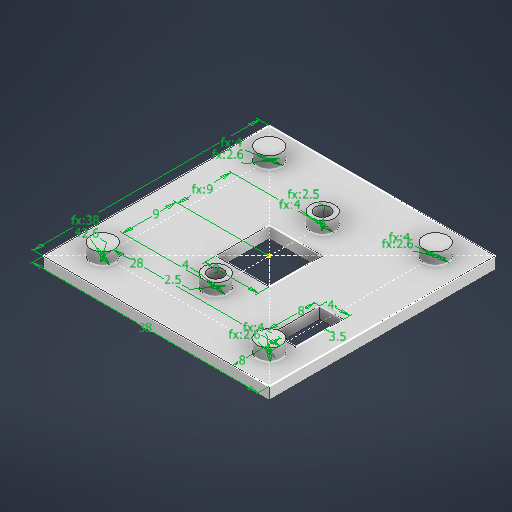
# Autodesk Inventor part: CameraMount
Saved by Autodesk Inventor 2025.1 (Build 291241000, 241)
## iProperties
Created: 2024-11-09
Part Number: CameraMount
Material: Generic
Document SubType Name: Modeling
Designer: jerem
Density: 1 g/cm^3
Appearance: Default
Author: jerem
## iProperties of the stored document CameraMount_3DPrint.ipt
Created: 2024-11-09
Part Number: CameraMount_3DPrint
Material: Generic
Document SubType Name: Modeling
Designer: jerem
Density: 1 g/cm^3
Appearance: Default
Author: jerem
Autodesk Inventor part; units mm, degrees
ref_plane "YZ Plane" through (0, 0, 0) normal (1, 0, 0) x (0, 1, 0)
ref_plane "XZ Plane" through (0, 0, 0) normal (0, 1, 0) x (-1, 0, 0)
ref_plane "XY Plane" through (0, 0, 0) normal (0, 0, 1) x (1, 0, 0)
sketch "Sketch1" plane through (0, 0, 0) normal (0, 1, 0) x (-1, 0, 0)
  line L0 (-19, -19) -> (19, -19)
  line L1 (19, -19) -> (19, 19)
  line L2 (19, 19) -> (-19, 19)
  line L3 (-19, 19) -> (-19, -19)
  line L4 (-19, -19) -> (19, 19) construction
  line L5 (19, -19) -> (-19, 19) construction
  line L6 (4.5, -4.5) -> (-4.5, -4.5)
  line L7 (-4.5, -4.5) -> (-4.5, 4.5)
  line L8 (-4.5, 4.5) -> (4.5, 4.5)
  line L9 (4.5, 4.5) -> (4.5, -4.5)
  line L10 (4.5, -4.5) -> (-4.5, 4.5) construction
  line L11 (-4.5, -4.5) -> (4.5, 4.5) construction
  circle A0 centre (14, 14) radius 1.3
  circle A1 centre (0, 9) radius 1.25
  circle A2 centre (-14, 14) radius 1.3
  circle A3 centre (0, -9) radius 1.25
  line L12 (0, 0) -> (0, 9) construction
  line L13 (0, -9) -> (0, 0) construction
  circle A4 centre (14, -14) radius 1.3
  circle A5 centre (-14, -14) radius 1.3
  line L14 (14, 14) -> (14, -14) construction
  line L15 (14, 14) -> (-14, 14) construction
  line L16 (-14, 14) -> (-14, -14) construction
  circle A6 centre (0, -9) radius 2
  circle A7 centre (0, 9) radius 2
  circle A8 centre (14, 14) radius 2
  circle A9 centre (-14, 14) radius 2
  circle A10 centre (-14, -14) radius 2
  circle A11 centre (14, -14) radius 2
  line L17 (-11.5, 3) -> (-15.5, 3)
  line L18 (-15.5, 3) -> (-15.5, 11)
  line L19 (-15.5, 11) -> (-11.5, 11)
  line L20 (-11.5, 11) -> (-11.5, 3)
  point P0 (0, 0)
  dimension "d0" = 38
  dimension "d1" = 38
  dimension "d2" = 9
  dimension "d3" = 2.5
  dimension "d4" = 2.5
  dimension "d5" = 9
  dimension "d6" = 9
  dimension "d7" = 2.6
  dimension "d8" = 2.6
  dimension "d9" = 2.6
  dimension "d10" = 2.6
  dimension "d11" = 28
  dimension "d14" = 4
  dimension "d15" = 4
  dimension "d16" = 4
  dimension "d17" = 4
  dimension "d18" = 4
  dimension "d19" = 4
  dimension "d20" = 8
  dimension "d21" = 4
  dimension "d22" = 8
  dimension "d23" = 3.5
  constraints: 43 end point, 12 centre point, 7 coincident, 6 parallel, 5 point on line, 4 horizontal, 4 midpoint, 4 vertical, 3 perpendicular
  measures "d0" distance of L3.start L4.end
  measures "d1" distance of L0.end L4.end
  measures "d2" distance of L7.end L8.end
  measures "d3" diameter of A1
  measures "d4" diameter of A3
  measures "d5" distance of L13.end L13.start
  measures "d6" distance of L13.end L12.end
  measures "d7" diameter of A0
  measures "d8" diameter of A4
  measures "d9" diameter of A2
  measures "d10" diameter of A5
  measures "d11" distance of L15.start L16.start
  measures "d14" diameter of A6
  measures "d15" diameter of A7
  measures "d16" diameter of A8
  measures "d17" diameter of A9
  measures "d18" diameter of A10
  measures "d19" diameter of A11
  measures "d20" distance of L19.end L17.start
  measures "d21" distance of L17.start L17.end
  measures "d22" distance between parallel lines of L2 L19
  measures "d23" distance between parallel lines of L3 L18
extrude "Extrusion1" add sketch "Sketch1" against normal blind 2 contours L3 L2 L1 L0 | A0 | A2 | A4 | A5 | A6 | A7 | A8 | A9 | A10 | A11
extrude "Extrusion2" add sketch "Sketch1" along normal blind 2 contours A0 | A2 | A4 | A5 | A6 | A7 | A8 | A9 | A10 | A11
equation "\"d1\" = d0"
equation "\"d4\" = d3"
equation "\"d5\" = d6"
equation "\"d8\" = d7"
equation "\"d9\" = d7"
equation "\"d10\" = d7"
equation "\"d14\" = d15"
equation "\"d17\" = d16"
equation "\"d18\" = d16"
equation "\"d19\" = d16"
body "Solid1"
